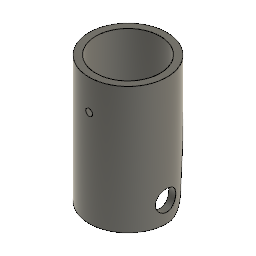
Suporte_Motor (Autodesk Fusion 360 design; units mm, degrees)
Autodesk Fusion 360 part; units mm, degrees
sketch "Esboço1" plane through (0, 0, 0) normal (0, 0, 1) x (1, 0, 0)
  circle A0 centre (0, 0) radius 19
  circle A1 centre (0, 0) radius 23
  dimension "d1" = 38
  dimension "d4" = 46
  constraint coincident A0.centre A1.centre
  measures "d1" diameter of A0
  measures "d4" diameter of A1
extrude "Extrusão1" add sketch "Esboço1" along normal blind 75
sketch "Esboço2" plane through (0, 0, 0) normal (1, 0, 0) x (0, 1, 0)
  line L0 (10.4842, -0.1929) -> (84.4879, -0.1929)
  arc A0 (23, 55.8071) -> (10.4842, -0.1929) centre (159.9133, -4.1911) ccw
  line L1 (23, 55.8071) -> (84.4879, -0.1929)
  line L2 (23, 75) -> (23, 43.6921) construction
  line L3 (23, 75) -> (-23, 75)
  dimension "d25" = 56
  constraint horizontal L0
  constraint coincident L0 A0.end
  constraint vertical L2
  constraint coincident L2.start L3.start
  constraint coincident A0.start L2
  measures "d25" distance of L0 A0.start
extrude "Extrusão2" cut sketch "Esboço2" along normal blind 40 and the other way blind 40
sketch "Esboço3" plane through (0, 0, 0) normal (0, 1, 0) x (1, 0, 0)
  circle A0 centre (0, -57) radius 2
  line L0 (0, 0) -> (0, -86.9144) construction
  dimension "d9" = 57
  dimension "d10" = 4
  constraint coincident L0.start origin
  constraint vertical L0
  constraint coincident A0.centre L0
  measures "d9" distance of L0.start A0.centre
  measures "d10" diameter of A0
extrude "Extrusão3" cut sketch "Esboço3" against normal blind 34
sketch "Esboço4" plane through (0, 0, 0) normal (1, 0, 0) x (0, 1, 0)
  line L0 (0, 0) -> (50.9154, 0) construction
  line L1 (0, 0) -> (0, 49.6753) construction
  circle A0 centre (0, 12) radius 6
  circle A1 centre (0, 12) radius 5.5
  dimension "d13" = 12
  dimension "d14" = 12
  dimension "d19" = 11
  constraint coincident L0.start L1.start
  constraint horizontal L0
  constraint perpendicular L0 L1
  constraint coincident L1 A0.centre
  constraint concentric A0 A1
  measures "d13" diameter of A0
  measures "d14" distance of L0.start A0.centre
  measures "d19" diameter of A1
extrude "Extrusão4" cut sketch "Esboço4" along normal blind 45 and the other way blind 35 contours A0 | A1
fillet "Arredondamento1" radius 10 2 edges at (18.1554, 10.4895, 0) (-18.1554, 10.4895, 0)
equation "d4 = d1 + 8 mm"
